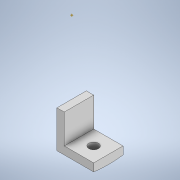
# Autodesk Inventor part: Slider_Winkel
Saved by Autodesk Inventor 2022.2 (Build 262287010, 287A)
## iProperties
Created: 2024-01-10
Part Number: Slider_Winkel
Material: Generisch
Document SubType Name: Modeling
Designer: ppovolni
Density: 1 g/cm^3
Appearance: Vorgabe
Author: ppovolni
Autodesk Inventor part; units mm, degrees
ref_plane "YZ Plane" through (0, 0, 0) normal (1, 0, 0) x (0, 1, 0)
ref_plane "XZ Plane" through (0, 0, 0) normal (0, 1, 0) x (-1, 0, 0)
ref_plane "XY Plane" through (0, 0, 0) normal (0, 0, 1) x (1, 0, 0)
sketch "Skizze1" plane through (0, 0, 0) normal (1, 0, 0) x (0, 1, 0)
  circle A0 centre (0, 0) radius 75.5 construction
  arc A1 (-74.8348, 10) -> (-74.8348, -10) centre (0, 0) ccw
  line L0 (-74.8348, 10) -> (-69.5, 10)
  line L1 (-69.5, 10) -> (-69.5, -10)
  line L2 (-69.5, -10) -> (-74.8348, -10)
  point P0 (-75.5, 0)
  dimension "d3" = 151
  dimension "d4" = 6
  dimension "d5" = 20
  constraints: 6 end point, 5 point on circle, 2 centre point, 2 perpendicular, 1 coincident, 1 concentric, 1 horizontal, 1 parallel
  measures "d3" diameter of A0
  measures "d4" distance from line of point (-75.5, 0) L1
  measures "d5" distance of L0.end L1.end
extrude "Extrusion1" add sketch "Skizze1" along normal blind 25
sketch "Skizze2" plane through (0, -69.5, 10) normal (0, 1, 0) x (1, 0, 0)
  line L0 (0, 0) -> (5, 0)
  line L1 (5, 0) -> (5, 20)
  line L2 (5, 20) -> (0, 20)
  line L3 (0, 20) -> (0, 0)
  line L4 (0, 20) -> (25, 20) projected
  point P0 (0, 10)
  dimension "d8" = 5
  constraints: 8 end point, 2 parallel, 1 collinear, 1 horizontal, 1 perpendicular
  measures "d8" distance between parallel lines of L1 L3
extrude "Extrusion2" add sketch "Skizze2" along normal blind 20
sketch "Skizze3" plane through (25, -69.5, 10) normal (0, 1, 0) x (1, 0, 0)
  circle A0 centre (-10, 10) radius 3.25
  line L0 (-20, 20) -> (-20, 0) construction
  line L1 (-20, 0) -> (0, 0) construction
  line L2 (0, 20) -> (0, 0) construction
  line L3 (-20, 20) -> (0, 20) construction
  line L4 (-20, 20) -> (0, 0) construction
  line L5 (0, 20) -> (-20, 0) construction
  point P0 (-25, 10)
  dimension "d11" = 6.5
  constraints: 4 end point, 2 midpoint, 1 centre point, 1 perpendicular
  measures "d11" diameter of A0
extrude "Extrusion4" cut sketch "Skizze3" against normal blind 10
